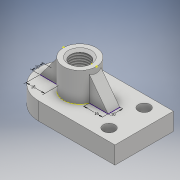
# Autodesk Inventor part: Основание дз курганова
Saved by Autodesk Inventor 2017 (Build 210142000, 142)
## iProperties
Part Number: Основание дз курганова
Material: Типовые
Document SubType Name: Modeling
Designer: Sasha
Density: 1 g/cm^3
Appearance: По умолчанию
Mass: 73.6369 g
Surface Area: 170.735 cm^2
Volume: 73.6369 cm^3
Author: Sasha
Autodesk Inventor part; units mm, degrees
ref_plane "YZ Plane" through (0, 0, 0) normal (1, 0, 0) x (0, 1, 0)
ref_plane "XY Plane" through (0, 0, 0) normal (0, 0, 1) x (1, 0, 0)
sketch "Эскиз1" plane through (0, 0, 0) normal (0, 0, 1) x (1, 0, 0)
  line L0 (-69.2132, 0) -> (64.0355, 0) projected
  line L1 (0, -42.2487) -> (0, 42.2487) projected
  line L2 (-20, 25) -> (45, 25)
  line L3 (45, 25) -> (45, -25)
  line L4 (45, -25) -> (-20, -25)
  line L5 (-45, 0) -> (-45, 0)
  arc A0 (-20, 25) -> (-45, 0) centre (-20, 0) ccw
  arc A1 (-45, 0) -> (-20, -25) centre (-20, 0) ccw
  point P0 (0, 0)
  point P1 (-45, 25)
  dimension "d0" = 50
  dimension "d1" = 90
  dimension "d2" = 25
  constraints: 8 end point, 4 point on circle, 4 tangent, 2 centre point, 2 parallel, 2 point on line, 1 concentric, 1 horizontal, 1 perpendicular, 2 other
  measures "d0" distance of L2.end L3.end
  measures "d1" distance of point (-45, 25) L2.end
  measures "d2" radius of A0
extrude "Выдавливание1" add sketch "Эскиз1" along normal blind 15
sketch "Эскиз2" plane through (0, 0, 15) normal (0, 0, 1) x (1, 0, 0)
  line L0 (45, -25) -> (45, 25) projected
  circle A0 centre (-10, 0) radius 14
  point P0 (0, 0)
  point P1 (30, 14.0013)
  point P2 (31.2898, -16.1928)
  dimension "d6" = 15
  dimension "d7" = 40
  dimension "d8" = 28
  constraints: 1 centre point, 1 coincident
  measures "d6" distance from line of L0 point (30, 14.001)
  measures "d7" horizontal distance of point (-10, 0) point (30, 14.001)
  measures "d8" diameter of A0
extrude "Выдавливание2" add sketch "Эскиз2" along normal blind 25
sketch "Эскиз3" plane through (-10, 0, 40) normal (0, 0, 1) x (1, 0, 0)
  point P0 (10, 0)
sketch "Эскиз4" plane through (-10, 0, 40) normal (0, 0, 1) x (1, 0, 0)
  point P0 (10, 0)
  point P1 (0, 0)
hole "Отверстие1" at (-10, 0, 40) direction (0, 0, -1) diameter 15.835 depth 30 thread size "M18x2" class "6H" standard "ISO Metric profile"
chamfer "Фаска1" distance 2 angle 45 1 edges at (-10, 7.9175, 40)
sketch "Эскиз5" plane through (0, 0, 15) normal (0, 0, 1) x (1, 0, 0)
  line L0 (45, -25) -> (45, 25) projected
  circle A0 centre (-10, 0) radius 7.9175 projected
  line L1 (-63, 0) -> (63, 0) projected
  line L2 (0, -35) -> (0, 35) projected
  point P0 (0, 0)
  point P1 (30, 15)
  point P2 (30, -15)
  dimension "d21" = 15
  dimension "d22" = 40
  dimension "d23" = 30
  constraints: 1 symmetric about line
  measures "d21" distance from line of L0 point (30, 15)
  measures "d22" horizontal distance of A0.centre point (30, 15)
  measures "d23" distance of point (30, -15) point (30, 15)
hole "Отверстие2" at (30, 15, 15) at (30, -15, 15) direction (0, 0, -1) diameter 10 end through all
sketch "Эскиз6" plane through (0, 0, 0) normal (0, 1, 0) x (-1, 0, 0)
  point P0 (0, 0)
sketch "Эскиз7" plane through (0, 0, 15) normal (0, 0, 1) x (1, 0, 0)
  line L0 (-39.0767, 5) -> (-23.0767, 5)
  line L1 (-23.0767, 5) -> (-23.0767, -5)
  line L2 (-23.0767, -5) -> (-39.0767, -5)
  line L3 (-39.0767, -5) -> (-39.0767, 5)
  circle A0 centre (-10, 0) radius 14 projected
  point P0 (0, 0)
  dimension "d31" = 10
  dimension "d32" = 16
  constraints: 8 end point, 2 parallel, 2 point on circle, 1 horizontal, 1 perpendicular
  measures "d31" distance of L2.end L0.start
  measures "d32" distance of L1.end L2.end
sketch "Эскиз8" plane through (0, 0, 0) normal (0, 1, 0) x (-1, 0, 0)
  line L0 (23.0767, 15) -> (39.0767, 15) projected
  line L1 (39.0767, 15) -> (24, 35)
  point P0 (0, 0)
  point P1 (24, 40)
  dimension "d33" = 5
  constraints: 2 end point, 1 vertical alignment
  measures "d33" distance of point (24, 40) L1.end
extrude "Ребро жесткости1" add sketch "Эскиз8" along normal mid plane 10 rib yes fills toward (31.0767, 15.05) open curves L0 L1
sketch "Эскиз9" plane through (0, 0, 15) normal (0, 0, 1) x (1, 0, 0)
  line L0 (3.0767, 5) -> (19.0767, 5)
  line L1 (19.0767, 5) -> (19.0767, -5)
  line L2 (19.0767, -5) -> (3.0767, -5)
  line L3 (3.0767, -5) -> (3.0767, 5)
  circle A0 centre (-10, 0) radius 14 projected
  point P0 (0, 0)
  dimension "d40" = 16
  dimension "d41" = 10
  constraints: 8 end point, 2 parallel, 2 point on circle, 1 horizontal, 1 perpendicular
  measures "d40" distance of L1.end L2.end
  measures "d41" distance of L0.end L1.end
sketch "Эскиз10" plane through (0, 0, 0) normal (0, 1, 0) x (-1, 0, 0)
  line L0 (-4, 35) -> (-19.0767, 15)
  point P0 (0, 0)
  point P1 (-4, 40)
  point P2 (-19.0767, 15)
  dimension "d42" = 5
  constraints: 2 end point, 1 coincident, 1 vertical alignment
  measures "d42" distance of point (-4, 40) L0.start
extrude "Ребро жесткости2" add sketch "Эскиз10" along normal mid plane 10 rib yes fills toward (-11.4984, 24.9699) open curves L0
